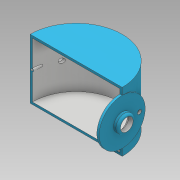
# Autodesk Inventor part: 헤드(하)
Saved by Autodesk Inventor 2018 (Build 220112000, 112)
## iProperties
Created: 2018-04-19
Part Number: 헤드(하)
Material: 일반
Document SubType Name: Modeling
Designer: CK
Density: 1 g/cm^3
Appearance: 기본값
Mass: 22.9944 g
Surface Area: 236.418 cm^2
Volume: 22.9944 cm^3
Author: CK
Autodesk Inventor part; units mm, degrees
ref_plane "XZ Plane" through (0, 0, 0) normal (0, 1, 0) x (-1, 0, 0)
ref_plane "XY Plane" through (0, 0, 0) normal (0, 0, 1) x (1, 0, 0)
sketch "스케치1" plane through (0, 0, 0) normal (0, 0, 1) x (1, 0, 0)
  arc A0 (40, 0) -> (-40, 0) centre (0, 0) ccw
  line L0 (-40, 0) -> (40, 0)
  dimension "d0" = 80
  constraints: 2 end point, 2 point on circle, 1 centre point, 1 coincident, 1 horizontal
  measures "d0" diameter of A0
extrude "돌출1" add sketch "스케치1" along normal mid plane 52
shell "쉘1" thickness 2 removed faces 1 at (13.3333, 0, 8.6667)
ref_plane "작업 평면1" through (40, 0, 0) normal (1, 0, 0) x (0, 1, 0)
sketch "스케치2" plane through (40, 0, 0) normal (1, 0, 0) x (0, 1, 0)
  line L0 (0, -26) -> (0, 26) projected
  arc A0 (0, 20) -> (0, -20) centre (0, 0) ccw
  line L1 (0, -20) -> (0, 20)
  dimension "d14" = 40
  constraints: 2 end point, 2 point on circle, 2 point on line, 1 centre point, 1 coincident, 1 collinear
  measures "d14" diameter of A0
extrude "돌출2" add sketch "스케치2" against normal blind 2
sketch "스케치6" plane through (40, 0, 0) normal (1, 0, 0) x (0, 1, 0)
  arc A0 (0, -20) -> (0, 20) centre (0, 0) ccw
  line L0 (0, -24) -> (0, 24) projected
  line L1 (0, -20) -> (0, 20)
  dimension "d15" = 40
  constraints: 2 end point, 2 point on circle, 2 point on line, 1 centre point, 1 coincident
  measures "d15" diameter of A0
extrude "돌출5" add sketch "스케치6" against normal up to surface
sketch "스케치7" plane through (40, 0, 0) normal (1, 0, 0) x (0, 0, -1)
  line L0 (31.2861, 15) -> (-52.9789, 15) construction
  line L1 (-20, 0) -> (20, 0) projected
  circle A0 centre (0, 15) radius 3.25
  point P0 (0, 0)
  dimension "d18" = 15
  dimension "d19" = 6.5
  constraints: 2 end point, 1 centre point, 1 horizontal, 1 point on line
  measures "d18" distance between parallel lines of L0 L1
  measures "d19" diameter of A0
extrude "돌출6" cut sketch "스케치7" against normal blind 10
sketch "스케치8" plane through (38, 0, 0) normal (-1, 0, 0) x (0, 0, 1)
  spline S0 degree 2 poles (-3.25, 15) (-3.25, 20.6292) (1.625, 17.8146) (6.5, 15) (1.625, 12.1854) (-3.25, 9.3708) (-3.25, 15) knots 0 0 0 0.333333 0.333333 0.666667 0.666667 1 1 1 weights 1 0.5 1 0.5 1 0.5 1 projected
  circle A0 centre (0, 15) radius 3.25 projected
  circle A1 centre (0, 15) radius 3.25
  circle A2 centre (0, 15) radius 4.5
  point P0 (0, 0)
  dimension "d22" = 9
  constraints: 2 centre point, 2 coincident, 1 vertical alignment, 1 other
  measures "d22" diameter of A2
extrude "돌출7" add sketch "스케치8" along normal blind 10
sketch "스케치13" plane through (40, 0, 0) normal (1, 0, 0) x (0, 0, -1)
  circle A0 centre (0, 15) radius 3.25 projected
  circle A1 centre (0, 15) radius 1.75
  circle A2 centre (0, 15) radius 3.25
  point P0 (0, 0)
  dimension "d35" = 3.5
  constraints: 2 centre point, 2 coincident, 1 concentric
  measures "d35" diameter of A1
extrude "돌출10" add sketch "스케치13" against normal blind 2
sketch "스케치14" plane through (28, 15, 0) normal (-1, 0, 0) x (0, 0, 1)
  line L0 (4.5, 0) -> (-4.5, 0)
  line L1 (-4.5, 0) -> (-4.5, 10)
  line L2 (-4.5, 10) -> (4.5, 10)
  line L3 (4.5, 10) -> (4.5, 0)
  arc A0 (4.5, 0) -> (-4.5, 0) centre (0, 0) ccw
  point P0 (0, -15)
  dimension "d38" = 10
  constraints: 8 end point, 2 parallel, 2 point on circle, 1 centre point, 1 coincident, 1 horizontal, 1 perpendicular
  measures "d38" distance of L0.end L1.end
extrude "돌출11" add sketch "스케치14" against normal up to surface contours A0 L1 L2 L3
sketch "스케치15" plane through (28, 0, 0) normal (-1, 0, 0) x (0, 0, 1)
  circle A0 centre (0, 19.8) radius 1.35
  arc A1 (-4.5, 15) -> (4.5, 15) centre (0, 15) ccw projected
  point P0 (0, 0)
  dimension "d41" = 2.7
  dimension "d42" = 4.8
  constraints: 1 centre point, 1 other
  measures "d41" diameter of A0
  measures "d42" distance of A1.centre A0.centre
extrude "돌출12" cut sketch "스케치15" against normal blind 6
sketch "스케치16" plane through (0, 0, 0) normal (1, 0, 0) x (0, 1, 0)
  circle A0 centre (19.8, 0) radius 2
  point P0 (0, 0)
  dimension "d45" = 4
  constraints: 1 centre point
  measures "d45" diameter of A0
extrude "돌출14" cut sketch "스케치16" against normal up to surface
sketch "스케치17" plane through (0, 0, 0) normal (0, 1, 0) x (-1, 0, 0)
  circle A0 centre (0, 0) radius 12.5
  dimension "d50" = 25
  constraints: 1 centre point, 1 coincident
  measures "d50" diameter of A0
extrude "돌출15" cut sketch "스케치17" along normal through all
sketch "스케치18" plane through (0, 0, 0) normal (0, 1, 0) x (-1, 0, 0)
  circle A0 centre (38.5, 0) radius 0.85
  line L0 (40, -26) -> (40, 26) projected
  point P0 (0, 0)
  point P1 (39.35, 0)
  dimension "d53" = 1.7
  dimension "d54" = 1.5
  constraints: 1 horizontal alignment, 2 other
  measures "d54" distance from line of L0 point (38.5, 0)
extrude "돌출16" cut sketch "스케치18" along normal up to surface
sketch "스케치19" plane through (-40, 0, 26) normal (0, -1, 0) x (1, 0, 0)
  arc A0 (2, -25.3126) -> (2, -26.6874) centre (1.5, -26) ccw projected
  arc A1 (1.5, -27.5) -> (1.5, -24.5) centre (1.5, -26) ccw
  line L0 (1.5, -27.5) -> (1.5, -24.5)
  arc A2 (1.5, -26.85) -> (1.5, -25.15) centre (1.5, -26) ccw
  point P0 (40, -26)
  dimension "d57" = 3
  constraints: 4 point on circle, 2 centre point, 2 coincident, 2 end point, 2 point on line, 1 vertical
  measures "d57" diameter of A1
extrude "돌출17" add sketch "스케치19" against normal blind 8 contours A0 L0 A1 A2
sketch "스케치21" plane through (40, 0, 0) normal (1, 0, 0) x (0, 0, -1)
  line L0 (-20, 0) -> (20, 0) projected
  circle A0 centre (0, 0) radius 7.5
  dimension "d62" = 15
  constraints: 1 centre point, 1 midpoint
  measures "d62" diameter of A0
extrude "돌출18" cut sketch "스케치21" against normal blind 6
sketch "스케치22" plane through (40, 0, 0) normal (1, 0, 0) x (0, 0, -1)
  circle A0 centre (0, 0) radius 7.5
  constraints: 1 centre point, 1 coincident
extrude "돌출19" add sketch "스케치22" along normal blind 4
fillet "모깎기1" radius 2 1 edges at (44, 0, 7.5)
sketch "스케치23" plane through (44, 0, 0) normal (1, 0, 0) x (0, 0, -1)
  circle A0 centre (0, 0) radius 5.5
  constraints: 1 centre point, 1 coincident
extrude "돌출20" cut sketch "스케치23" against normal blind 4
